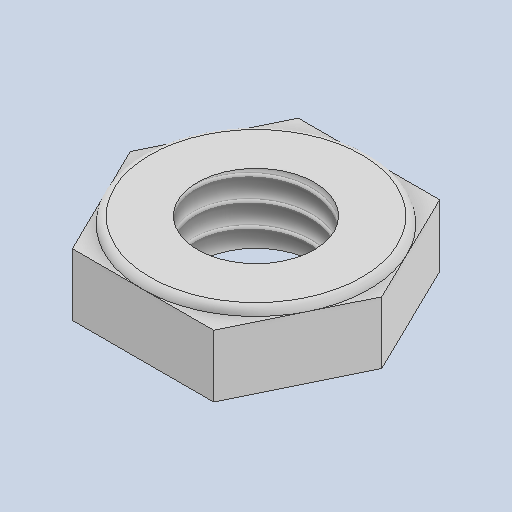
# Autodesk Inventor part: nakretka_CPY
Saved by Autodesk Inventor 2025.2 (Build 292293000, 293)
## iProperties
Created: 2025-03-26
Part Number: nakretka_CPY
Material: Ogólny
Document SubType Name: Modeling
Designer: tadek
Density: 1 g/cm^3
Appearance: Domyślna
Author: tadek
Autodesk Inventor part; units mm, degrees
ref_plane "YZ Plane" through (0, 0, 0) normal (1, 0, 0) x (0, 1, 0)
ref_plane "XZ Plane" through (0, 0, 0) normal (0, 1, 0) x (-1, 0, 0)
ref_plane "XY Plane" through (0, 0, 0) normal (0, 0, 1) x (1, 0, 0)
sketch "Szkic1" plane through (0, 0, 0) normal (0, 1, 0) x (-1, 0, 0)
  circle A0 centre (0, 0) radius 2.5
  line L0 (0, 0) -> (0, -4)
  line L1 (0, 0) -> (0, 4)
  circle A1 centre (0, 0) radius 4
  line L2 (5.4643, 0) -> (-5.9483, 0)
  line L3 (0, 4) -> (2.5, 4)
  line L4 (0, 4) -> (-2.5, 4)
  line L5 (2.5, 4) -> (3.5955, 1.7528)
  line L6 (3.5955, 1.7528) -> (4.45, 0)
  line L7 (4.45, 0) -> (3.5955, -1.7528)
  line L8 (3.5955, -1.7528) -> (2.5, -4)
  line L9 (2.5, -4) -> (0, -4)
  line L10 (0, -4) -> (-2.5, -4)
  line L11 (-2.5, 4) -> (-3.5955, 1.7528)
  line L12 (-3.5955, 1.7528) -> (-4.45, 0)
  line L13 (-2.5, -4) -> (-4.45, 0)
  point P0 (-3.5955, -1.7528)
  dimension "d0" = 5
  dimension "d1" = 4
  dimension "d2" = 4
  dimension "d3" = 8
  dimension "d4" = 2.5
  dimension "d5" = 2.5
  constraints: 28 end point, 7 point on line, 7 tangent, 3 point on circle, 2 centre point, 2 coincident, 2 horizontal, 2 vertical
  measures "d0" diameter of A0
  measures "d1" distance of L0.start L0.end
  measures "d2" distance of L0.start L1.end
  measures "d3" diameter of A1
  measures "d4" distance of L1.end L3.end
  measures "d5" distance of L1.end L4.end
extrude "Wyciągnięcie proste2" add sketch "Szkic1" along normal blind 2.2 contours L2 L7 A1 | A1 L6 L2 | L3 L5 A1 | A1 L11 L4 | L10 L13 A1 | A1 L8 L9 | L2 L12 A1 | A1 L13 L2
extrude "Wyciągnięcie proste3" add sketch "Szkic1" along normal blind 2.45 contours L2 L1 A0 | L2 A1 L0 A0 | A0 L1 A1 L2 | A0 L0 L2 | L1 L2 A0 | A0 L2 A1 L1 | L0 A1 L2 A0 | A0 L2 L0
sketch "Szkic2" plane through (0, 2.45, 0) normal (0, 1, 0) x (1, 0, 0)
  point P0 (0, 0)
  point P1 (0, 0)
  constraints: 1 coincident
hole "Otwór1" at (0, 2.45, 0) at (0, 2.45, 0) direction (0, -1, 0) diameter 4.134 depth 14.2 tip angle 118 thread size "M5x0.8" class "6H" standard "ANSI Metric M Profile"
fillet "Zaokrąglenie1" radius 0.25 1 edges at (4, 2.45, 0)
